y_pulley_holder_front (Autodesk Fusion 360 design; units mm, degrees)
Autodesk Fusion 360 part; units mm, degrees
sketch "Sketch1" plane through (0, 0, 0) normal (0, 1, 0) x (1, 0, 0)
  line L0 (0, 0) -> (50, 0)
  line L1 (50, 0) -> (50, -30)
  line L2 (50, -30) -> (0, -30)
  line L3 (0, -30) -> (0, 0)
  circle A0 centre (5.5, -15) radius 1.6
  circle A1 centre (44.5, -15) radius 1.6
  circle A2 centre (25, -21.15) radius 2.1
  point P0 (25, -21.15)
  dimension "d1" = 30
  dimension "d2" = 50
  dimension "d3" = 15
  dimension "d4" = 5.5
  dimension "d5" = 5.5
  dimension "d6" = 3.2
  dimension "d9" = 25
  dimension "d10" = 21.15
  dimension "d19" = 4.2
  constraint horizontal L0
  constraint vertical L1
  constraint horizontal L2
  constraint vertical L3
  constraint coincident L0.start L3.end
  constraint horizontal A0.centre A1.centre
  constraint equal A0 A1
  constraint coincident P0 A2.centre
  measures "d1" distance of L0.start L2.end
  measures "d2" distance of L1.end L2.end
  measures "d3" distance of L0 A0.centre
  measures "d4" distance of L3 A0.centre
  measures "d5" distance of L1 A1.centre
  measures "d6" diameter of A0
  measures "d9" distance of L3 P0
  measures "d10" distance of L0 P0
  measures "d19" diameter of A2
extrude "Extrude1" add sketch "Sketch1" against normal blind 5
sketch "Sketch2" plane through (0, -5, 0) normal (0, -1, 0) x (1, 0, 0)
  circle A0 centre (44.5, 15) radius 1.6
  circle A1 centre (5.5, 15) radius 1.6
  line L0 (50, 30) -> (0, 30)
  line L1 (0, 30) -> (0, 0)
  line L2 (0, 0) -> (50, 0)
  line L3 (50, 0) -> (50, 30)
  line L4 (33.75, 33.4) -> (16.25, 33.4)
  line L5 (16.25, 33.4) -> (16.25, 8.9)
  line L6 (16.25, 8.9) -> (33.75, 8.9)
  line L7 (33.75, 8.9) -> (33.75, 33.4)
  line L8 (33.75, 33.4) -> (16.25, 8.9) construction
  line L9 (16.25, 33.4) -> (33.75, 8.9) construction
  circle A2 centre (25, 21.15) radius 2.1
  line L10 (29.75, 12.9) -> (20.25, 12.9)
  line L11 (20.25, 12.9) -> (20.25, 29.4)
  line L12 (20.25, 29.4) -> (29.75, 29.4)
  line L13 (29.75, 29.4) -> (29.75, 12.9)
  line L14 (29.75, 12.9) -> (20.25, 29.4) construction
  line L15 (20.25, 12.9) -> (29.75, 29.4) construction
  point P0 (25, 21.15)
  point P1 (25, 21.15)
  dimension "d20" = 16.5
  dimension "d21" = 9.5
  dimension "d22" = 4
  dimension "d23" = 4
  constraint horizontal L4
  constraint perpendicular L4 L5
  constraint parallel L4 L6
  constraint parallel L5 L7
  constraint coincident L8 P1
  constraint coincident L9 P1
  constraint midpoint L8 P1
  constraint horizontal L10
  constraint perpendicular L10 L11
  constraint parallel L10 L12
  constraint parallel L11 L13
  constraint coincident L14 P1
  constraint coincident L15 P1
  constraint coincident P1 P0
  measures "d20" distance of L10.end L11.end
  measures "d21" distance of L10.start L10.end
  measures "d22" distance of L5 L11
  measures "d23" distance of L4 L12
extrude "Extrude2" add sketch "Sketch2" along normal blind 14 and the other way up to surface (5 mm away) contours L0 L5 L6 L7 | L0 L4 L5 L7
extrude "Extrude3" cut 1 faces at (25.0523, -5, 14.952) along direction (0, 1, 0) blind 2
sketch "Sketch3" plane through (0, 0, 0) normal (0, 1, 0) x (-1, 0, 0)
  circle A0 centre (-5.5, 15) radius 1.6
  circle A1 centre (-44.5, 15) radius 1.6
  line L0 (-33.75, 30) -> (-50, 30)
  line L1 (-50, 30) -> (-50, 0)
  line L2 (-50, 0) -> (0, 0)
  line L3 (0, 0) -> (0, 30)
  line L4 (0, 30) -> (-16.25, 30)
  line L5 (-16.25, 30) -> (-16.25, 33.4)
  line L6 (-16.25, 33.4) -> (-33.75, 33.4)
  line L7 (-33.75, 33.4) -> (-33.75, 30)
  circle A2 centre (-25, 21.15) radius 2.1
  circle A3 centre (-44.5, 7) radius 3
  circle A4 centre (-5.5, 7) radius 3
  dimension "d28" = 6
  dimension "d32" = 8
  constraint vertical A1.centre A3.centre
  constraint vertical A0.centre A4.centre
  constraint horizontal A3.centre A4.centre
  constraint equal A3 A4
  measures "d28" diameter of A3
  measures "d32" distance of A1.centre A3.centre
extrude "Extrude4" cut sketch "Sketch3" against normal blind 3 contours A3 | A4
chamfer "Chamfer1" distance 8.9 angle 45 3 edges at (16.25, -5, 19.45) (33.75, -5, 19.45) (25, -5, 8.9)
chamfer "Chamfer3" distance 4 angle 45 2 edges at (33.75, -9.5, 33.4) (16.25, -9.5, 33.4)
fillet "Fillet2" radius 3 10 edges at (0, -2.5, 30) (0, -2.5, 0) (50, -2.5, 30) (50, -2.5, 0) (33.75, -16.45, 8.9) (16.25, -16.45, 8.9) (16.25, -16.45, 29.4) (20.25, -9.5, 33.4) (29.75, -9.5, 33.4) (33.75, -16.45, 29.4)
equation "d3 = d1 / 2"
equation "d5 = d4"
equation "d9 = d2 / 2"
equation "d10 = ( 42.3 / 2 ) * 1 mm"
equation "d23 = d22"
